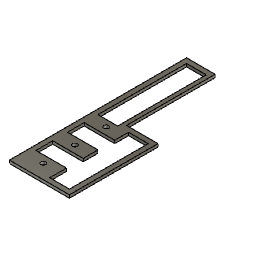
TV Cabinet Rack Posts (Autodesk Fusion 360 design; units mm, degrees)
Autodesk Fusion 360 part; units mm, degrees
sketch "Sketch1" plane through (0, 0, 0) normal (0, 0, 1) x (1, 0, 0) in component "Top-RIght-Front2"
  line L0 (0, 0) -> (-20, 0)
  line L1 (-20, 0) -> (-20, -180)
  line L2 (-20, -180) -> (0, -180)
  line L3 (0, -180) -> (0, 0)
  dimension "d41" = 20
  dimension "d42" = 180
  constraint horizontal L0
  constraint vertical L1
  constraint horizontal L2
  constraint vertical L3
  constraint coincident L0.start L3.end
  measures "d41" distance of L0.start L0.end
  measures "d42" distance of L0.start L2.end
sketch "Sketch2" plane through (0, 0, 0) normal (0, 0, 1) x (1, 0, 0) in component "Top-RIght-Front2"
  line L0 (0, 0) -> (9, 0)
  line L1 (9, 0) -> (9, -180)
  line L2 (9, -180) -> (0, -180)
  line L3 (0, -180) -> (0, 0)
  dimension "d43" = 9
  dimension "d44" = 180
  constraint horizontal L0
  constraint vertical L1
  constraint horizontal L2
  constraint vertical L3
  constraint coincident L0.start L3.end
  measures "d43" distance of L0.start L0.end
  measures "d44" distance of L0.start L2.end
extrude "Extrude1" add sketch "Sketch1" sketch "Sketch2" along normal blind 3 of sketch 2 in component "Top-RIght-Front2"
sketch "Sketch3" plane through (0, 0, 3) normal (0, 0, 1) x (-1, 0, 0) in component "Top-RIght-Front2"
  line L0 (-9, 0) -> (20, 0)
  line L1 (20, 0) -> (20, 180)
  line L2 (20, 180) -> (-9, 180)
  line L3 (-9, 180) -> (-9, 0)
  line L4 (0, 0) -> (0, 270) construction
  circle A0 centre (0, 101.5) radius 2.5
  dimension "d47" = 270
  dimension "d48" = 5
  dimension "d49" = 101.5
  constraint coincident L4.start origin
  constraint perpendicular L2 L4
  constraint coincident L4 A0.centre
  measures "d47" distance of L4.start L4.end
  measures "d48" diameter of A0
  measures "d49" distance of L4.start A0.centre
extrude "Extrude2" cut sketch "Sketch3" against normal up to surface (3 mm away) contours A0 in component "Top-RIght-Front2"
sketch "Sketch5" plane through (0, 0, 3) normal (0, 0, 1) x (-1, 0, 0) in component "Top-RIght-Front2"
  circle A0 centre (0, 101.5) radius 2.5
  line L0 (-9, 0) -> (20, 0)
  line L1 (20, 0) -> (20, 180)
  line L2 (20, 180) -> (-9, 180)
  line L3 (-9, 180) -> (-9, 0)
  line L4 (0, 0) -> (0, 226.7762) construction
  circle A1 centre (0, 133.5) radius 2.5
  circle A2 centre (0, 165.5) radius 2.5
  dimension "d52" = 5
  dimension "d53" = 32
  dimension "d54" = 5
  dimension "d55" = 32
  constraint coincident L4.start origin
  constraint perpendicular L0 L4
  constraint coincident L4 A1.centre
  constraint coincident L4 A2.centre
  measures "d52" diameter of A1
  measures "d53" distance of A0.centre A1.centre
  measures "d54" diameter of A2
  measures "d55" distance of A1.centre A2.centre
extrude "Extrude3" cut sketch "Sketch5" against normal up to surface (3 mm away) contours A1 | A2 in component "Top-RIght-Front2"
sketch "Sketch10" plane through (0, 0, 3) normal (0, 0, 1) x (-1, 0, 0) in component "Top-RIght-Front2"
  circle A0 centre (0, 133.5) radius 2.5
  circle A1 centre (0, 165.5) radius 2.5
  circle A2 centre (0, 101.5) radius 2.5
  line L0 (-9, 0) -> (20, 0)
  line L1 (20, 0) -> (20, 180)
  line L2 (20, 180) -> (-9, 180)
  line L3 (-9, 180) -> (-9, 0)
  line L4 (-9, 90) -> (-41, 90)
  line L5 (-41, 90) -> (-41, 180)
  line L6 (-41, 180) -> (-9, 180)
  line L7 (-9, 180) -> (-9, 90)
  dimension "d82" = 32
  dimension "d83" = 90
  constraint horizontal L4
  constraint vertical L5
  constraint horizontal L6
  constraint vertical L7
  constraint coincident L3 L4.start
  constraint collinear L2 L6
  measures "d82" distance of L4.start L4.end
  measures "d83" distance of L4.start L2.end
extrude "Extrude6" add sketch "Sketch10" against normal up to surface (3 mm away) contours L3 L4 L5 L6 L7 in component "Top-RIght-Front2"
sketch "Sketch11" plane through (0, 0, 3) normal (0, 0, 1) x (-1, 0, 0) in component "Top-RIght-Front2"
  circle A0 centre (0, 133.5) radius 2.5
  circle A1 centre (0, 165.5) radius 2.5
  circle A2 centre (0, 101.5) radius 2.5
  line L0 (-9, 0) -> (20, 0)
  line L1 (20, 0) -> (20, 180)
  line L2 (20, 180) -> (-41, 180)
  line L3 (-41, 180) -> (-41, 90)
  line L4 (-41, 90) -> (-9, 90)
  line L5 (-9, 90) -> (-9, 0)
  line L6 (15, 5) -> (-5, 5)
  line L7 (-5, 5) -> (-5, 95)
  line L8 (-5, 95) -> (15, 95)
  line L9 (15, 95) -> (15, 5)
  line L10 (-16, 95) -> (-36, 95)
  line L11 (-36, 95) -> (-36, 175)
  line L12 (-36, 175) -> (-16, 175)
  line L13 (-16, 175) -> (-16, 95)
  line L14 (-16, 109) -> (15, 109)
  line L15 (15, 109) -> (15, 126)
  line L16 (15, 126) -> (-16, 126)
  line L17 (-16, 126) -> (-16, 109)
  line L18 (-16, 141) -> (15, 141)
  line L19 (15, 141) -> (15, 158)
  line L20 (15, 158) -> (-16, 158)
  line L21 (-16, 158) -> (-16, 141)
  dimension "d86" = 20
  dimension "d87" = 90
  dimension "d88" = 5
  dimension "d89" = 5
  dimension "d90" = 20
  dimension "d91" = 80
  dimension "d92" = 5
  dimension "d93" = 5
  dimension "d94" = 31
  dimension "d95" = 17
  dimension "d96" = 7.5
  dimension "d97" = 31
  dimension "d98" = 17
  dimension "d99" = 7.5
  constraint horizontal L6
  constraint vertical L7
  constraint horizontal L8
  constraint vertical L9
  constraint horizontal L10
  constraint vertical L11
  constraint horizontal L12
  constraint vertical L13
  constraint horizontal L14
  constraint vertical L15
  constraint horizontal L16
  constraint vertical L17
  constraint coincident L13 L14.start
  constraint horizontal L18
  constraint vertical L19
  constraint horizontal L20
  constraint vertical L21
  constraint coincident L13 L18.start
  measures "d86" distance of L6.start L6.end
  measures "d87" distance of L6.start L8.end
  measures "d88" distance of L0 L6
  measures "d89" distance of L1 L9
  measures "d90" distance of L10.start L10.end
  measures "d91" distance of L10.start L12.end
  measures "d92" distance of L4 L10
  measures "d93" distance of L3 L11
  measures "d94" distance of L14.start L14.end
  measures "d95" distance of L14.start L16.end
  measures "d96" distance of A2.centre L14
  measures "d97" distance of L18.start L18.end
  measures "d98" distance of L18.start L20.end
  measures "d99" distance of A0.centre L18
extrude "Extrude7" cut sketch "Sketch11" against normal up to surface (3 mm away) contours L6 L7 L8 L9 | L10 L11 L12 L13 L17 L21 | L13 L14 L15 L16 L17 | L13 L18 L19 L20 L21 in component "Top-RIght-Front2"
component "Top-RIght-Front2" placed x (1, 0, 0) y (0, 1, 0) z (0, 0, 1) at (0, 0, 0)
